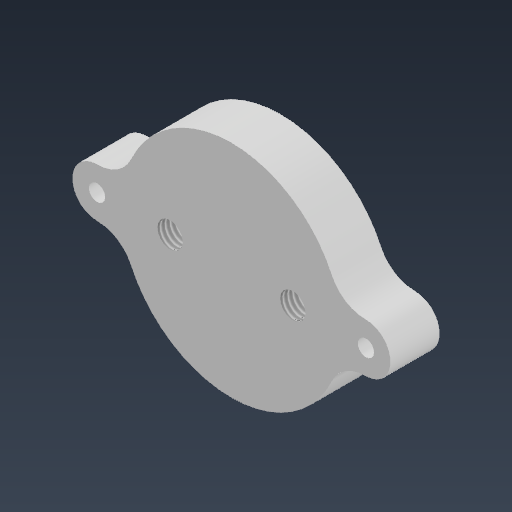
# Autodesk Inventor part: extruder waterblock
Saved by Autodesk Inventor 2024.3 (Build 283343000, 343)
## iProperties
Created: 2024-09-28
Part Number: extruder waterblock
Material: Generic
Document SubType Name: Modeling
Designer: MFil
Density: 1 g/cm^3
Appearance: Default
Author: MFil
Autodesk Inventor part; units mm, degrees
ref_plane "YZ Plane" through (0, 0, 0) normal (1, 0, 0) x (0, 1, 0)
ref_plane "XZ Plane" through (0, 0, 0) normal (0, 1, 0) x (-1, 0, 0)
ref_plane "XY Plane" through (0, 0, 0) normal (0, 0, 1) x (1, 0, 0)
sketch "Sketch1" plane through (0, 0, 0) normal (0, 0, 1) x (1, 0, 0)
  circle A0 centre (0, -18.1) radius 17.9 projected
  circle A1 centre (0, -18.1) radius 2.9 projected
  circle A2 centre (-13.5, -18.1) radius 1.525 projected
  circle A3 centre (13.5, -18.1) radius 1.525 projected
  circle A4 centre (0, -18.1) radius 18
  arc A5 (23.0705, -21.2782) -> (23.0705, -14.9218) centre (21.92, -18.1) ccw projected
  line L0 (23.0705, -14.9218) -> (17.5529, -12.9245) projected
  arc A6 (17.5529, -23.2755) -> (17.5529, -12.9245) centre (0, -18.1) ccw projected
  line L1 (17.5529, -23.2755) -> (23.0705, -21.2782) projected
  circle A7 centre (21.92, -18.1) radius 1.325 projected
  arc A8 (-23.0705, -14.9218) -> (-23.0705, -21.2782) centre (-21.92, -18.1) ccw projected
  line L2 (-23.0705, -21.2782) -> (-17.5529, -23.2755) projected
  arc A9 (-17.5529, -12.9245) -> (-17.5529, -23.2755) centre (0, -18.1) ccw projected
  line L3 (-17.5529, -12.9245) -> (-23.0705, -14.9218) projected
  circle A10 centre (-21.92, -18.1) radius 1.325 projected
  line L4 (0, -18.1) -> (-21.92, -18.1)
  line L5 (-21.92, -18.1) -> (21.92, -18.1)
  circle A11 centre (21.92, -18.1) radius 4
  circle A12 centre (-21.92, -18.1) radius 4
  circle A13 centre (21.8177, -28.0995) radius 6
  circle A14 centre (21.8177, -8.1005) radius 6
  circle A15 centre (-21.8177, -28.0995) radius 6
  circle A16 centre (-21.8177, -8.1005) radius 6
  point P0 (0, 0)
  point P1 (16.3632, -25.5996)
  point P2 (21.8791, -22.0998)
  point P3 (21.8791, -14.1002)
  point P4 (16.3632, -10.6004)
  point P5 (-16.3632, -10.6004)
  point P6 (-21.8791, -14.1002)
  point P7 (-21.8791, -22.0998)
  point P8 (-16.3632, -25.5996)
  dimension "d0" = 36
  dimension "d1" = 8
  dimension "d2" = 8
  dimension "d3" = 12
  dimension "d4" = 12
  dimension "d5" = 12
  dimension "d6" = 12
  constraints: 8 tangent, 7 centre point, 4 end point, 3 coincident, 1 collinear, 1 horizontal
  measures "d0" diameter of A4
  measures "d1" diameter of A11
  measures "d2" diameter of A12
  measures "d3" diameter of A13
  measures "d4" diameter of A14
  measures "d5" diameter of A16
  measures "d6" diameter of A15
extrude "Extrusion1" add sketch "Sketch1" along normal blind 8 contours L5 A3 A1 L4 A2 A0 | L5 A11 A4 A12 L4 A0 | A0 L4 A2 A1 L5 A3 | A0 L4 A12 A4 A11 L5 | L5 A3 | A3 L5 | A11 A4 L5 | L5 A4 A11 | L4 A2 | A2 L4 | A12 A4 L4 | L4 A4 A12 | L5 A6 A11 A4 | A4 A11 A6 L5 | A4 A14 L0 A6 A11 | A11 A6 L1 A13 A4 | L4 A9 A12 A4 | A4 A12 A9 L4 | A12 A9 L3 A16 A4 | A4 A15 L2 A9 A12 | L5 L4 A1 | A1 L4 L5 | A6 A11 L0 A5 L1 | A6 L0 A14 A11 | A11 L1 A13 A6 | A9 A12 L2 A8 L3 | A12 L3 A16 A9 | A9 L2 A15 A12 | A11 L1 A5 L0 | L0 A14 A11 | A11 A13 L1 | A12 A16 L3 | L3 A8 L2 A12 | L2 A15 A12
sketch "Sketch2" plane through (0, 0, 8) normal (0, 0, 1) x (1, 0, 0)
  circle A0 centre (21.92, -18.1) radius 1.325 projected
  circle A1 centre (-21.92, -18.1) radius 1.325 projected
  line L0 (21.92, -18.1) -> (-21.92, -18.1)
  line L1 (0, -18.1) -> (-10, -18.1)
  line L2 (0, -18.1) -> (10, -18.1)
  point P0 (0, 0)
  dimension "d9" = 10
  dimension "d10" = 10
  constraints: 6 end point, 2 point on line, 1 horizontal, 1 midpoint
  measures "d9" distance of L1.start L1.end
  measures "d10" distance of L1.start L2.end
hole "Hole1" at (10, -18.1, 8) at (-10, -18.1, 8) direction (0, 0, -1) diameter 4.134 depth 4 thread size "M5x0.8" class "6H" standard "ISO Metric profile"
body "Solid1"
